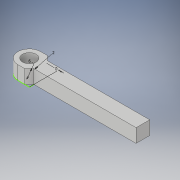
# Autodesk Inventor part: roka1
Saved by Autodesk Inventor 2019 (Build 230136000, 136)
## iProperties
Created: 2020-07-24
Part Number: roka1
Material: Generic
Document SubType Name: Modeling
Designer: lukad
Mass: 1.06197 g
Surface Area: 9.07277 cm^2
Volume: 1.06197 cm^3
Density: 1 g/cm^3
Appearance: Default
Author: lukad
Autodesk Inventor part; units mm, degrees
ref_plane "YZ Plane" through (0, 0, 0) normal (1, 0, 0) x (0, 1, 0)
ref_plane "XZ Plane" through (0, 0, 0) normal (0, 1, 0) x (-1, 0, 0)
ref_plane "XY Plane" through (0, 0, 0) normal (0, 0, 1) x (1, 0, 0)
sketch "Sketch1" plane through (0, 0, 0) normal (0, 1, 0) x (-1, 0, 0)
  circle A0 centre (-3.9982, 7.6265) radius 3
  circle A1 centre (-3.9982, 7.6265) radius 5
  line L0 (-3.9982, 12.6265) -> (-8.9982, 12.6265)
  line L1 (-8.9982, 12.6265) -> (-8.9982, 2.6265)
  line L2 (-8.9982, 2.6265) -> (-3.9982, 2.6265)
  line L3 (-3.9982, 2.6265) -> (-3.9982, 12.6265)
  point P0 (0, 0)
  dimension "d0" = 6
  dimension "d1" = 2
  dimension "d8" = 0
  constraints: 8 end point, 3 horizontal, 2 parallel, 1 centre point, 1 coincident, 1 perpendicular, 1 vertical alignment, 2 other
  measures "d0" diameter of A0
  measures "d8" horizontal extent of L1
extrude "Extrusion1" add sketch "Sketch1" along normal blind 6 contours A0 L3 A1 | A0 L3 A1
extrude "Extrusion2" add sketch "Sketch1" along normal blind 6 contours L3 A0 | A0 L3 A1 | A1 L1 L0 | L2 L1 A1 picked at (-5.8933, 7.7284) picked at (-4.3691, 3.335)
extrude "Extrusion3" cut sketch "Sketch1" along normal blind 6 contours A0 L3 | L3 A0
sketch "Sketch2" plane through (8.9982, 0, 12.6265) normal (1, 0, 0) x (0, 0, -1)
  line L0 (0, 0) -> (10, 0) projected
  line L1 (2, 6) -> (8, 6)
  line L2 (8, 6) -> (8, 0)
  line L3 (8, 0) -> (2, 0)
  line L4 (2, 0) -> (2, 6)
  line L5 (0, 0) -> (0, 6) projected
  line L6 (10, 0) -> (10, 6) projected
  line L7 (0, 6) -> (10, 6) projected
  point P0 (12.6265, 0)
  dimension "d9" = 2
  dimension "d10" = 2
  constraints: 8 end point, 2 parallel, 1 collinear, 1 horizontal, 1 perpendicular, 1 point on line
  measures "d9" distance between parallel lines of L4 L5
  measures "d10" distance between parallel lines of L6 L2
extrude "Extrusion4" add sketch "Sketch2" along normal blind 45 contours L4 L1 L2 L0
chamfer "Chamfer1" distance 2 angle 45 2 edges at (8.9982, 3, 12.6265) (8.9982, 3, 2.6265)
body "Solid1"
